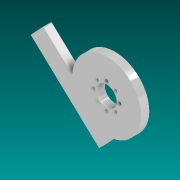
# Autodesk Inventor part: gearboxFrame
Saved by Autodesk Inventor 2020.2 (Build 242310000, 310)
## iProperties
Created: 2020-05-19
Part Number: gearboxFrame
Material: Aluminum 6061
Document SubType Name: Modeling
Designer: Svend
Density: 2.7 g/cm^3
Appearance: Aluminum - Polished
Author: Svend
Autodesk Inventor part; units mm, degrees
ref_plane "YZ Plane" through (0, 0, 0) normal (1, 0, 0) x (0, 1, 0)
ref_plane "XZ Plane" through (0, 0, 0) normal (0, 1, 0) x (-1, 0, 0)
ref_plane "Work Plane1" through (0, 0, 0) normal (0, 0, 1) x (1, 0, 0)
sketch "Sketch1" plane through (0, 0, 0) normal (0, 0, 1) x (1, 0, 0)
  circle A0 centre (0, 0) radius 12.5 projected
  circle A1 centre (0, -16) radius 2 projected
  circle A2 centre (0, 16) radius 2 projected
  circle A3 centre (-16, 0) radius 2 projected
  circle A4 centre (16, 0) radius 2 projected
  circle A5 centre (11.3137, 11.3137) radius 1.6 projected
  circle A6 centre (-11.3137, -11.3137) radius 1.6 projected
  circle A7 centre (-11.3137, 11.3137) radius 1.6 projected
  circle A8 centre (11.3137, -11.3137) radius 1.6 projected
  circle A9 centre (0, 0) radius 20.7 projected
  line L0 (31.6375, -97.9493) -> (-99.8575, 24.9697) projected
  line L1 (-23.1886, -46.699) -> (-9.2531, -59.7257) projected
  line L2 (15.1663, -37.3207) -> (23.5338, -32.6958) projected
  line L3 (34.2063, -21.2786) -> (38.2573, -12.6186) projected
  line L4 (40.1807, 2.8912) -> (38.3679, 12.2784) projected
  line L5 (30.8075, 25.9567) -> (23.8232, 32.4855) projected
  line L6 (9.6668, 39.1076) -> (0.1789, 40.2842) projected
  line L7 (-15.1663, 37.3207) -> (-23.5338, 32.6958) projected
  line L8 (-34.2063, 21.2786) -> (-38.2573, 12.6186) projected
  line L9 (-45.0314, -26.2807) -> (-35.471, -16.0534) projected
  line L10 (-28.404, -15.8151) -> (-13.8665, -29.4045) projected
  line L11 (-13.6283, -36.4716) -> (-23.1886, -46.699) projected
  circle A10 centre (33.3141, 1.123) radius 2.5 projected
  circle A11 centre (1.123, -33.3141) radius 2.5 projected
  circle A12 centre (0, 0) radius 21 projected
  circle A13 centre (-1.123, 33.3141) radius 2.5 projected
  circle A14 centre (-33.3141, -1.123) radius 2.5 projected
  arc A15 (-15.924, -38.9274) -> (-37.7667, -18.5092) centre (0, 0) ccw
  arc A16 (-28.404, -15.8151) -> (-35.471, -16.0534) centre (-31.8184, -19.4678) ccw
  arc A17 (-13.6283, -36.4716) -> (-13.8665, -29.4045) centre (-17.2809, -33.0572) ccw
  arc A18 (-77.068, 33.987) -> (-78.4814, 33.9394) centre (-77.7509, 33.2565) ccw projected
  line L12 (-78.4814, 33.9394) -> (-92.9244, 18.4887) projected
  line L13 (-92.9244, 18.4887) -> (-45.0314, -26.2807) projected
  arc A19 (-28.404, -15.8151) -> (-35.471, -16.0534) centre (-31.8184, -19.4678) ccw projected
  arc A20 (-13.6283, -36.4716) -> (-13.8665, -29.4045) centre (-17.2809, -33.0572) ccw projected
  line L14 (-9.2531, -59.7257) -> (9.7389, -39.4086) projected
  arc A21 (10.6702, -38.8458) -> (9.7389, -39.4086) centre (11.2, -40.7744) ccw projected
  arc A22 (10.6702, -38.8458) -> (15.1663, -37.3207) centre (0, 0) ccw projected
  arc A23 (23.5338, -32.6958) -> (34.2063, -21.2786) centre (0, 0) ccw projected
  arc A24 (38.2573, -12.6186) -> (40.1807, 2.8912) centre (0, 0) ccw projected
  arc A25 (38.3679, 12.2784) -> (30.8075, 25.9567) centre (0, 0) ccw projected
  arc A26 (23.8232, 32.4855) -> (9.6668, 39.1076) centre (0, 0) ccw projected
  arc A27 (0.1789, 40.2842) -> (-15.1663, 37.3207) centre (0, 0) ccw projected
  arc A28 (-23.5338, 32.6958) -> (-34.2063, 21.2786) centre (0, 0) ccw projected
  arc A29 (-38.2573, 12.6186) -> (-40.1013, 3.8394) centre (0, 0) ccw projected
  arc A30 (-43.4579, 2.5689) -> (-40.1013, 3.8394) centre (-42.0921, 4.03) ccw projected
  line L15 (-43.4579, 2.5689) -> (-77.068, 33.987) projected
  point P0 (0, 0)
  point P1 (7.9751, -41.2954)
  point P2 (36.8098, 20.3458)
  point P3 (-58.967, -13.254)
  point P4 (30.7249, -28.721)
  point P5 (30.7249, -28.721)
  point P6 (7.9751, -41.2954)
  point P7 (41.7388, -5.1762)
  point P8 (41.7388, -5.1762)
  point P9 (-41.7388, 5.1762)
  point P10 (-30.7249, 28.721)
  point P11 (-30.7249, 28.721)
  point P12 (17.8208, 38.0964)
  point P13 (17.8208, 38.0964)
  point P14 (-7.9751, 41.2954)
  point P15 (-7.9751, 41.2954)
  point P16 (7.9751, -41.2954)
  point P17 (-42.0094, 2.0317)
  constraints: 7 point on circle, 4 tangent, 3 centre point, 2 point on line, 1 coincident
extrude "Extrusion1" add sketch "Sketch1" along normal blind 10 contours A9 | L0 L11 A15 L14 | L0 L9 A16 L10 A17 L11 | L14 A21 A22 L2 A23 L3 A24 L4 A25 L5 A26 L6 A27 L7 A28 L8 A29 A30 A15 | A15 L11 A17 L10 A16 L9 A30 A29 L8 A28 L7 A27 L6 A26 L5 A25 L4 A24 L3 A23 L2 A22 A21 L14 | L0 L12 A18 L15 A30 A15 L9 | A10 | A11 | A12 | A13 | A14
sketch "Sketch2" plane through (-45.0314, -26.2807, 0) normal (-0.6828833, -0.7305275, 0) x (0.7305275, -0.6828833, 0)
  line L0 (-65.5595, 0) -> (48.976, 0) projected
  line L1 (-65.5595, 10) -> (48.976, 10) projected
  line L2 (-65.5595, 0) -> (48.976, 0) projected
  line L3 (48.976, 0) -> (48.976, 10) projected
  line L4 (-65.5595, 10) -> (48.976, 10) projected
  line L5 (-65.5595, 0) -> (-65.5595, 10) projected
  line L6 (48.976, 0) -> (48.976, 10) projected
  line L7 (-65.5595, 0) -> (-65.5595, 10) projected
  point P0 (14.95, 0)
  point P1 (-11.576, 5)
  point P2 (41.476, 5)
  point P3 (-19.076, 5)
  point P4 (29.9, 5)
  point P5 (-8.2917, 10)
  dimension "d10" = 7.5
  constraints: 2 horizontal alignment, 1 midpoint
  measures "d10" distance from line of L3 point (41.476, 5)
hole "Hole1" at (-53.488, -18.3757, 5) at (-14.732, -54.604, 5) direction (0.6828833, 0.7305275, 0) diameter 4.917 depth 17.1 tip angle 118 thread size "M6x1" class "6H" standard "ISO Metric profile"
sketch "Sketch3" plane through (0, 0, 10) normal (0, 0, 1) x (1, 0, 0)
  line L0 (-76.3375, 33.3041) -> (-73.606, 36.2263) projected
  line L1 (-48.5774, 7.3546) -> (-76.3375, 33.3041) projected
  line L2 (-45.8459, 10.2767) -> (-48.5774, 7.3546) projected
  line L3 (-45.8459, 10.2767) -> (-73.606, 36.2263) projected
  line L4 (-92.9244, 18.4887) -> (-9.2531, -59.7257) projected
  circle A0 centre (11.3137, -11.3137) radius 1.6 projected
  circle A1 centre (11.3137, 11.3137) radius 1.6 projected
  circle A2 centre (16, 0) radius 2 projected
  circle A3 centre (-16, 0) radius 2 projected
  circle A4 centre (-11.3137, -11.3137) radius 1.6 projected
  circle A5 centre (-11.3137, 11.3137) radius 1.6 projected
  circle A6 centre (0, 16) radius 2 projected
  circle A7 centre (0, -16) radius 2 projected
  circle A8 centre (0, 0) radius 12.5 projected
  line L5 (-41.7388, 5.1762) -> (-58.967, -13.254) projected
  line L6 (31.6375, -97.9493) -> (-99.8575, 24.9697) projected
  line L7 (-75.067, 37.592) -> (-92.9244, 18.4887)
  line L8 (-77.7985, 34.6699) -> (-47.1164, 5.9888)
  line L9 (-47.1164, 5.9888) -> (-43.8411, 2.9271)
  arc A9 (7.9751, -41.2954) -> (-42.0094, 2.0317) centre (0, 0) ccw projected
  arc A10 (-43.4579, 2.5689) -> (-42.0094, 2.0317) centre (-42.0921, 4.03) ccw projected
  line L10 (-43.4579, 2.5689) -> (-77.068, 33.987) projected
  arc A11 (-77.068, 33.987) -> (-78.4814, 33.9394) centre (-77.7509, 33.2565) ccw projected
  line L11 (-78.4814, 33.9394) -> (-92.9244, 18.4887) projected
  line L12 (-9.2531, -59.7257) -> (7.9751, -41.2954) projected
  point P0 (0, 0)
  point P1 (-44.3849, 8.9109)
  point P2 (-45.0314, -26.2807)
  point P3 (-23.1886, -46.699)
  constraints: 6 end point, 2 perpendicular, 2 point on line, 4 other
extrude "Extrusion2" [suppressed]
equation "\"d10\" = d9"
equation "\"d9\" = 7.5"
body "Solid1"
